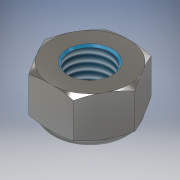
# Autodesk Inventor part: Nylon Insert Lock Nut M5
Saved by Autodesk Inventor 2019 (Build 230136000, 136)
## iProperties
Created: 2020-11-22
Part Number: Nylon Insert Lock Nut M5
Material: Steel
Document SubType Name: Modeling
Designer: asus
Density: 7.85 g/cm^3
Appearance: Chrome - Polished
Author: asus
Autodesk Inventor part; units mm, degrees
ref_plane "YZ Plane" through (0, 0, 0) normal (1, 0, 0) x (0, 1, 0)
ref_plane "XZ Plane" through (0, 0, 0) normal (0, 1, 0) x (-1, 0, 0)
ref_plane "XY Plane" through (0, 0, 0) normal (0, 0, 1) x (1, 0, 0)
sketch "Sketch1" plane through (0, 0, 0) normal (0, 1, 0) x (-1, 0, 0)
  circle A0 centre (0, 0) radius 3.17
  circle A1 centre (0, 0) radius 2.65
  circle A2 centre (0, 0) radius 2.125
  line L0 (0.0063, 4) -> (-2.3031, 4.0036)
  line L1 (2.3157, 3.9964) -> (0.0063, 4)
  arc A3 (3.4673, 1.9945) -> (0.0063, 4) centre (0, 0) ccw
  line L2 (3.4673, 1.9945) -> (2.3157, 3.9964)
  line L3 (4.6188, -0.0073) -> (3.4673, 1.9945)
  arc A4 (3.4609, -2.0055) -> (3.4673, 1.9945) centre (0, 0) ccw
  line L4 (3.4609, -2.0055) -> (4.6188, -0.0073)
  arc A5 (-0.0063, -4) -> (3.4609, -2.0055) centre (0, 0) ccw
  line L5 (2.3031, -4.0036) -> (3.4609, -2.0055)
  line L6 (-0.0063, -4) -> (2.3031, -4.0036)
  arc A6 (-3.4673, -1.9945) -> (-0.0063, -4) centre (0, 0) ccw
  line L7 (-2.3157, -3.9964) -> (-0.0063, -4)
  line L8 (-3.4673, -1.9945) -> (-2.3157, -3.9964)
  line L9 (-4.6188, 0.0073) -> (-3.4673, -1.9945)
  arc A7 (-3.4609, 2.0055) -> (-3.4673, -1.9945) centre (0, 0) ccw
  line L10 (-3.4609, 2.0055) -> (-4.6188, 0.0073)
  arc A8 (0.0063, 4) -> (-3.4609, 2.0055) centre (0, 0) ccw
  line L11 (-2.3031, 4.0036) -> (-3.4609, 2.0055)
  constraints: 24 end point, 12 point on circle, 9 centre point
extrude "Extrusion1" add sketch "Sketch1" along normal blind 4.17 contours A0 | A1 | A8 L11 L0 | L1 L2 A3 | A3 A4 A5 A6 A7 A8 | L3 L4 A4 | A7 L9 L10 | L5 L6 A5 | A6 L7 L8
extrude "Extrusion2" add sketch "Sketch1" against normal blind 0.83 contours A0 | A3 A4 A5 A6 A7 A8
extrude "Extrusion3" add sketch "Sketch1" against normal blind 0.6 contours A1
fillet "Fillet1" radius 0.83 1 edges at (3.4609, -0.83, 2.0055)
thread "Thread1" size "M4.5x0.75" class "6H" standard "ANSI Metric M Profile" full length
sketch "Sketch2" plane through (0, 0, 0) normal (0, 0, 1) x (1, 0, 0)
  line L0 (-4.6188, 0) -> (-3.4673, 0) projected
  line L1 (-4.6188, 0) -> (-4.6188, 4.17) projected
  line L2 (-4.6188, 4.17) -> (-2.3157, 4.17) projected
  line L3 (2.3157, 0) -> (0.0063, 0) projected
  line L4 (0.0063, 0) -> (0.0063, 2.976)
  line L5 (-4.6188, 0.289) -> (-3.999, 0)
  line L6 (-4.6188, 3.881) -> (-3.999, 4.17)
  line L7 (-2.3031, 4.17) -> (-4.6188, 4.17) projected
  line L8 (-3.999, 4.17) -> (-4.6188, 4.17)
  line L9 (-4.6188, 3.881) -> (-4.6188, 4.17)
  line L10 (-4.6188, 0.289) -> (-4.6188, 0)
  line L11 (-3.4609, 0) -> (-4.6188, 0) projected
  line L12 (-3.999, 0) -> (-4.6188, 0)
  point P0 (0, 0)
  dimension "d10" = 0.289
  dimension "d11" = 0.289
  dimension "d14" = 65
  dimension "d15" = 65
  constraints: 14 end point, 4 point on line, 3 collinear, 1 horizontal, 1 vertical
  measures "d10" distance from line of L0 L5.start
  measures "d11" distance from line of L2 L6.start
  measures "d14" angle of L5 L1
  measures "d15" angle of L6 L1
revolve "Revolution1" cut sketch "Sketch2" angle 360 about axis through (0.0063, 0, 0) along (0, 1, 0)
chamfer "Chamfer1" distance 0.2 angle 45 2 edges at (2.125, 4.17, 0) (2.125, -0.6, 0)
body "Solid1"
